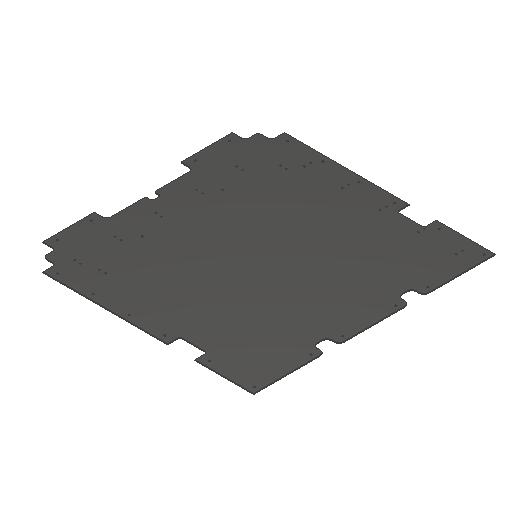
# Autodesk Inventor part: LC_PLEXI_2mm_Side_Wall_Back
Saved by Autodesk Inventor 2026.1 (Build 301233000, 233)
## iProperties
Created: 2016-06-26
Part Number: LC_PLEXI_2mm_Side_Wall_Back
Material: Ogólny
Document SubType Name: Modeling
Designer: Andrzej
Density: 1 g/cm^3
Appearance: Smooth - Black
Mass: 602.344 g
Surface Area: 6069.03 cm^2
Volume: 602.344 cm^3
Author: Andrzej
Autodesk Inventor part; units mm, degrees
ref_plane "YZ Plane" through (0, 0, 0) normal (1, 0, 0) x (0, 1, 0)
ref_plane "XZ Plane" through (0, 0, 0) normal (0, 1, 0) x (-1, 0, 0)
ref_plane "XY Plane" through (0, 0, 0) normal (0, 0, 1) x (1, 0, 0)
sketch "Szkic1" plane through (0, 0, 0) normal (0, 0, 1) x (1, 0, 0)
  line L0 (4.403, -85.7889) -> (549.403, -85.7889)
  line L1 (549.403, -85.7889) -> (549.403, -641.7889)
  line L2 (549.403, -641.7889) -> (4.403, -641.7889)
  line L3 (4.403, -641.7889) -> (4.403, -85.7889)
  line L4 (549.403, -477.9559) -> (521.403, -477.9559)
  line L5 (521.403, -477.9559) -> (521.403, -444.9559)
  line L6 (521.403, -444.9559) -> (549.403, -444.9559)
  line L7 (549.403, -444.9559) -> (549.403, -477.9559)
  line L8 (549.403, -282.6219) -> (521.403, -282.6219)
  line L9 (521.403, -282.6219) -> (521.403, -249.6219)
  line L10 (521.403, -249.6219) -> (549.403, -249.6219)
  line L11 (549.403, -249.6219) -> (549.403, -282.6219)
  line L12 (64.403, -641.7889) -> (64.403, -611.7889)
  line L13 (64.403, -611.7889) -> (34.403, -611.7889)
  line L14 (34.403, -611.7889) -> (34.403, -581.7889)
  line L15 (34.403, -581.7889) -> (4.403, -581.7889)
  line L16 (4.403, -145.7889) -> (34.403, -145.7889)
  line L17 (34.403, -145.7889) -> (34.403, -115.7889)
  line L18 (34.403, -115.7889) -> (64.403, -115.7889)
  line L19 (64.403, -115.7889) -> (64.403, -85.7889)
  line L20 (351.403, -641.7889) -> (414.403, -641.7889)
  line L21 (414.403, -641.7889) -> (414.403, -613.2889)
  line L22 (414.403, -613.2889) -> (351.403, -613.2889)
  line L23 (351.403, -613.2889) -> (351.403, -641.7889)
  line L24 (351.403, -85.7889) -> (414.403, -85.7889)
  line L25 (414.403, -85.7889) -> (414.403, -114.2889)
  line L26 (414.403, -114.2889) -> (351.403, -114.2889)
  line L27 (351.403, -114.2889) -> (351.403, -85.7889)
  line L28 (4.403, -463.7889) -> (32.903, -463.7889)
  line L29 (32.903, -463.7889) -> (32.903, -263.7889)
  line L30 (32.903, -263.7889) -> (4.403, -263.7889)
  line L31 (4.403, -263.7889) -> (4.403, -463.7889)
  line L32 (631.7363, -282.6219) -> (603.7363, -282.6219)
  line L33 (714.0696, -282.6219) -> (686.0696, -282.6219)
  line L34 (32.903, -373.7889) -> (47.903, -373.7889)
  line L35 (47.903, -373.7889) -> (47.903, -353.7889)
  line L36 (47.903, -353.7889) -> (32.903, -353.7889)
  point P0 (0, 0)
  point P1 (331.403, -628.2889)
  point P2 (84.403, -628.2889)
  point P3 (84.403, -99.2889)
  point P4 (331.403, -99.2889)
  point P5 (537.903, -628.2889)
  point P6 (434.403, -628.2889)
  point P7 (537.903, -497.9559)
  point P8 (537.903, -424.9559)
  point P9 (537.903, -302.6219)
  point P10 (537.903, -229.6219)
  point P11 (537.903, -99.2889)
  point P12 (434.403, -99.2889)
  point P13 (17.903, -561.7889)
  point P14 (17.903, -483.7889)
  point P15 (17.903, -243.7889)
  point P16 (17.903, -165.7889)
  point P17 (166.7363, -628.2889)
  point P18 (249.0696, -628.2889)
  point P19 (166.7363, -99.2889)
  point P20 (249.0696, -99.2889)
  point P21 (107.903, -456.4556)
  point P22 (107.903, -271.1223)
  dimension "d0" = 545
  dimension "d1" = 556
  dimension "d4" = 28
  dimension "d5" = 33
  dimension "d6" = 28
  dimension "d7" = 33
  dimension "d8" = 163.833
  dimension "d9" = 163.833
  dimension "d13" = 30
  dimension "d14" = 30
  dimension "d15" = 30
  dimension "d16" = 30
  dimension "d17" = 30
  dimension "d18" = 30
  dimension "d19" = 30
  dimension "d20" = 30
  dimension "d22" = 63
  dimension "d23" = 28.5
  dimension "d24" = 63
  dimension "d25" = 28.5
  dimension "d26" = 347
  dimension "d27" = 347
  dimension "d29" = 28.5
  dimension "d30" = 200
  dimension "d31" = 178
  dimension "d33" = 20
  dimension "d34" = 13.5
  dimension "d35" = 13.5
  dimension "d36" = 13.5
  dimension "d37" = 13.5
  dimension "d38" = 11.5
  dimension "d39" = 11.5
  dimension "d40" = 11.5
  dimension "d41" = 11.5
  dimension "d42" = 11.5
  dimension "d43" = 11.5
  dimension "d44" = 13.5
  dimension "d45" = 13.5
  dimension "d46" = 13.5
  dimension "d47" = 13.5
  dimension "d48" = 13.5
  dimension "d49" = 13.5
  dimension "d50" = 13.5
  dimension "d51" = 13.5
  dimension "d52" = 20
  dimension "d53" = 20
  dimension "d54" = 20
  dimension "d55" = 20
  dimension "d56" = 20
  dimension "d57" = 20
  dimension "d58" = 20
  dimension "d59" = 20
  dimension "d60" = 20
  dimension "d61" = 20
  dimension "d62" = 20
  dimension "d63" = 20
  dimension "d64" = 20
  dimension "d65" = 247
  dimension "d68" = 82.3333
  dimension "d75" = 82.3333
  dimension "d87" = 103.5
  dimension "d88" = 103.5
  dimension "d89" = 185.3333
  dimension "d90" = 185.3333
  constraints: 74 end point, 14 perpendicular, 12 parallel, 11 point on line, 10 horizontal, 1 vertical, 10 other
  measures "d0" distance of L1.end L2.end
  measures "d1" distance of L0.end L1.end
  measures "d4" distance of L5.end L6.end
  measures "d5" distance of L4.end L5.end
  measures "d6" distance of L9.end L10.end
  measures "d7" distance of L8.end L9.end
  measures "d8" distance between parallel lines of L2 L4
  measures "d9" distance between parallel lines of L0 L10
  measures "d13" distance of L12.start L12.end
  measures "d14" distance of L12.end L13.end
  measures "d15" distance of L13.end L14.end
  measures "d16" distance of L14.end L15.end
  measures "d17" distance of L16.start L16.end
  measures "d18" distance of L16.end L17.end
  measures "d19" distance of L17.end L18.end
  measures "d20" distance of L18.end L19.end
  measures "d22" distance between parallel lines of L21 L23
  measures "d23" distance between parallel lines of L20 L22
  measures "d24" distance of L25.end L26.end
  measures "d25" distance of L24.end L25.end
  measures "d26" distance between parallel lines of L3 L23
  measures "d27" distance between parallel lines of L3 L27
  measures "d29" distance of L30.end L29.end
  measures "d30" distance of L29.end L28.end
  measures "d31" distance between parallel lines of L2 L28
  measures "d33" distance from line of L12 point (84.403, -628.289)
  measures "d34" distance from line of L2 point (84.403, -628.289)
  measures "d35" distance from line of L2 point (331.403, -628.289)
  measures "d36" distance from line of L2 point (434.403, -628.289)
  measures "d37" distance from line of L2 point (537.903, -628.289)
  measures "d38" distance from line of L1 point (537.903, -628.289)
  measures "d39" distance from line of L1 point (537.903, -497.956)
  measures "d40" distance from line of L1 point (537.903, -424.956)
  measures "d41" distance from line of L1 point (537.903, -302.622)
  measures "d42" distance from line of L1 point (537.903, -229.622)
  measures "d43" distance from line of L1 point (537.903, -99.289)
  measures "d44" distance from line of L0 point (537.903, -99.289)
  measures "d45" distance from line of L0 point (434.403, -99.289)
  measures "d46" distance from line of L0 point (331.403, -99.289)
  measures "d47" distance from line of L0 point (84.403, -99.289)
  measures "d48" distance from line of L3 point (17.903, -165.789)
  measures "d49" distance from line of L3 point (17.903, -243.789)
  measures "d50" distance from line of L3 point (17.903, -483.789)
  measures "d51" distance from line of L3 point (17.903, -561.789)
  measures "d52" distance from line of L28 point (17.903, -483.789)
  measures "d53" distance from line of L15 point (17.903, -561.789)
  measures "d54" distance from line of L30 point (17.903, -243.789)
  measures "d55" distance from line of L16 point (17.903, -165.789)
  measures "d56" distance from line of L19 point (84.403, -99.289)
  measures "d57" distance from line of L27 point (331.403, -99.289)
  measures "d58" distance from line of L25 point (434.403, -99.289)
  measures "d59" distance from line of L10 point (537.903, -229.622)
  measures "d60" distance from line of L8 point (537.903, -302.622)
  measures "d61" distance from line of L6 point (537.903, -424.956)
  measures "d62" distance from line of L4 point (537.903, -497.956)
  measures "d63" distance from line of L21 point (434.403, -628.289)
  measures "d64" distance from line of L23 point (331.403, -628.289)
  measures "d65" distance of point (331.403, -628.289) point (84.403, -628.289)
  measures "d68" distance of L8.start L32.start
  measures "d75" distance of point (84.403, -99.289) point (166.736, -99.289)
  measures "d87" distance from line of point (107.903, -456.456) L3
  measures "d88" distance from line of L3 point (107.903, -271.122)
  measures "d89" distance from line of L2 point (107.903, -456.456)
  measures "d90" distance from line of L0 point (107.903, -271.122)
extrude "Wyciągnięcie proste1" add sketch "Szkic1" along normal blind 2
extrude "Wyciągnięcie proste2" cut sketch "Szkic1" along normal blind 2 contours L0 L19 L18 L17 L16 L3 | L0 L25 L26 L27 | L30 L29 L28 L3 | L15 L14 L13 L12 L2 L3 | L36 L35 L34 L29 | L1 L8 L9 L10 | L1 L4 L5 L6 | L23 L22 L21 L2
fillet "Zaokrąglenie1" radius 10 8 edges at (549.403, -477.9559, 1) (521.403, -477.9559, 1) (521.403, -444.9559, 1) (549.403, -444.9559, 1) (549.403, -282.6219, 1) (521.403, -282.6219, 1) (521.403, -249.6219, 1) (549.403, -249.6219, 1)
fillet "Zaokrąglenie2" radius 8 6 edges at (34.403, -581.7889, 1) (34.403, -611.7889, 1) (64.403, -611.7889, 1) (34.403, -145.7889, 1) (34.403, -115.7889, 1) (64.403, -115.7889, 1)
fillet "Zaokrąglenie3" radius 5 4 edges at (351.403, -613.2889, 1) (414.403, -613.2889, 1) (351.403, -114.2889, 1) (414.403, -114.2889, 1)
fillet "Zaokrąglenie4" radius 10 2 edges at (32.903, -463.7889, 1) (32.903, -263.7889, 1)
hole "Otwór1" at (331.403, -628.2889, 0) at (84.403, -628.2889, 0) at (84.403, -99.2889, 0) at (331.403, -99.2889, 0) at (537.903, -628.2889, 0) at (434.403, -628.2889, 0) at (537.903, -497.9559, 0) at (537.903, -424.9559, 0) at (537.903, -302.6219, 0) at (537.903, -229.6219, 0) at (537.903, -99.2889, 0) at (434.403, -99.2889, 0) at (17.903, -561.7889, 0) at (17.903, -483.7889, 0) at (17.903, -243.7889, 0) at (17.903, -165.7889, 0) at (166.7363, -628.2889, 0) at (249.0696, -628.2889, 0) at (166.7363, -99.2889, 0) at (249.0696, -99.2889, 0) at (107.903, -456.4556, 0) at (107.903, -271.1223, 0) direction (0, 0, 1) diameter 4 end through all
fillet "Zaokrąglenie5" radius 4 4 edges at (32.903, -373.7889, 1) (47.903, -373.7889, 1) (47.903, -353.7889, 1) (32.903, -353.7889, 1)
sketch "Szkic2" plane through (0, 0, 0) normal (0, 0, -1) x (-1, 0, 0)
  circle A0 centre (-107.903, -456.4556) radius 2 projected
  circle A1 centre (-166.7363, -99.2889) radius 2 projected
  circle A2 centre (-166.7363, -628.2889) radius 2 projected
  circle A3 centre (-17.903, -243.7889) radius 2 projected
  circle A4 centre (-17.903, -561.7889) radius 2 projected
  circle A5 centre (-537.903, -99.2889) radius 2 projected
  circle A6 centre (-537.903, -302.6219) radius 2 projected
  circle A7 centre (-537.903, -497.9559) radius 2 projected
  circle A8 centre (-537.903, -628.2889) radius 2 projected
  circle A9 centre (-84.403, -99.2889) radius 2 projected
  circle A10 centre (-331.403, -628.2889) radius 2 projected
  circle A11 centre (-84.403, -628.2889) radius 2 projected
  circle A12 centre (-331.403, -99.2889) radius 2 projected
  circle A13 centre (-434.403, -628.2889) radius 2 projected
  circle A14 centre (-537.903, -424.9559) radius 2 projected
  circle A15 centre (-537.903, -229.6219) radius 2 projected
  circle A16 centre (-434.403, -99.2889) radius 2 projected
  circle A17 centre (-17.903, -483.7889) radius 2 projected
  circle A18 centre (-17.903, -165.7889) radius 2 projected
  circle A19 centre (-249.0696, -628.2889) radius 2 projected
  circle A20 centre (-249.0696, -99.2889) radius 2 projected
  circle A21 centre (-107.903, -271.1223) radius 2 projected
  arc A22 (-36.903, -353.7889) -> (-32.903, -349.7889) centre (-36.903, -349.7889) ccw projected
  line L0 (-32.903, -349.7889) -> (-32.903, -273.7889) projected
  arc A23 (-22.903, -263.7889) -> (-32.903, -273.7889) centre (-22.903, -273.7889) ccw projected
  line L1 (-22.903, -263.7889) -> (-4.403, -263.7889) projected
  line L2 (-4.403, -263.7889) -> (-4.403, -145.7889) projected
  line L3 (-4.403, -145.7889) -> (-26.403, -145.7889) projected
  arc A24 (-34.403, -137.7889) -> (-26.403, -145.7889) centre (-26.403, -137.7889) ccw projected
  line L4 (-34.403, -137.7889) -> (-34.403, -123.7889) projected
  arc A25 (-34.403, -123.7889) -> (-42.403, -115.7889) centre (-42.403, -123.7889) ccw projected
  line L5 (-42.403, -115.7889) -> (-56.403, -115.7889) projected
  arc A26 (-64.403, -107.7889) -> (-56.403, -115.7889) centre (-56.403, -107.7889) ccw projected
  line L6 (-64.403, -107.7889) -> (-64.403, -85.7889) projected
  line L7 (-64.403, -85.7889) -> (-351.403, -85.7889) projected
  line L8 (-351.403, -85.7889) -> (-351.403, -109.2889) projected
  arc A27 (-356.403, -114.2889) -> (-351.403, -109.2889) centre (-356.403, -109.2889) ccw projected
  line L9 (-356.403, -114.2889) -> (-409.403, -114.2889) projected
  arc A28 (-414.403, -109.2889) -> (-409.403, -114.2889) centre (-409.403, -109.2889) ccw projected
  line L10 (-414.403, -109.2889) -> (-414.403, -85.7889) projected
  line L11 (-414.403, -85.7889) -> (-549.403, -85.7889) projected
  line L12 (-549.403, -85.7889) -> (-549.403, -239.6219) projected
  arc A29 (-549.403, -239.6219) -> (-539.403, -249.6219) centre (-539.403, -239.6219) ccw projected
  line L13 (-539.403, -249.6219) -> (-531.403, -249.6219) projected
  arc A30 (-521.403, -259.6219) -> (-531.403, -249.6219) centre (-531.403, -259.6219) ccw projected
  line L14 (-521.403, -259.6219) -> (-521.403, -272.6219) projected
  arc A31 (-531.403, -282.6219) -> (-521.403, -272.6219) centre (-531.403, -272.6219) ccw projected
  line L15 (-531.403, -282.6219) -> (-539.403, -282.6219) projected
  arc A32 (-539.403, -282.6219) -> (-549.403, -292.6219) centre (-539.403, -292.6219) ccw projected
  line L16 (-549.403, -292.6219) -> (-549.403, -434.9559) projected
  arc A33 (-549.403, -434.9559) -> (-539.403, -444.9559) centre (-539.403, -434.9559) ccw projected
  line L17 (-539.403, -444.9559) -> (-531.403, -444.9559) projected
  arc A34 (-521.403, -454.9559) -> (-531.403, -444.9559) centre (-531.403, -454.9559) ccw projected
  line L18 (-521.403, -454.9559) -> (-521.403, -467.9559) projected
  arc A35 (-531.403, -477.9559) -> (-521.403, -467.9559) centre (-531.403, -467.9559) ccw projected
  line L19 (-531.403, -477.9559) -> (-539.403, -477.9559) projected
  arc A36 (-539.403, -477.9559) -> (-549.403, -487.9559) centre (-539.403, -487.9559) ccw projected
  line L20 (-549.403, -487.9559) -> (-549.403, -641.7889) projected
  line L21 (-549.403, -641.7889) -> (-414.403, -641.7889) projected
  line L22 (-414.403, -641.7889) -> (-414.403, -618.2889) projected
  arc A37 (-409.403, -613.2889) -> (-414.403, -618.2889) centre (-409.403, -618.2889) ccw projected
  line L23 (-409.403, -613.2889) -> (-356.403, -613.2889) projected
  arc A38 (-351.403, -618.2889) -> (-356.403, -613.2889) centre (-356.403, -618.2889) ccw projected
  line L24 (-351.403, -618.2889) -> (-351.403, -641.7889) projected
  line L25 (-351.403, -641.7889) -> (-64.403, -641.7889) projected
  line L26 (-64.403, -641.7889) -> (-64.403, -619.7889) projected
  arc A39 (-56.403, -611.7889) -> (-64.403, -619.7889) centre (-56.403, -619.7889) ccw projected
  line L27 (-56.403, -611.7889) -> (-42.403, -611.7889) projected
  arc A40 (-42.403, -611.7889) -> (-34.403, -603.7889) centre (-42.403, -603.7889) ccw projected
  line L28 (-34.403, -603.7889) -> (-34.403, -589.7889) projected
  arc A41 (-26.403, -581.7889) -> (-34.403, -589.7889) centre (-26.403, -589.7889) ccw projected
  line L29 (-26.403, -581.7889) -> (-4.403, -581.7889) projected
  line L30 (-4.403, -581.7889) -> (-4.403, -463.7889) projected
  line L31 (-4.403, -463.7889) -> (-22.903, -463.7889) projected
  arc A42 (-32.903, -453.7889) -> (-22.903, -463.7889) centre (-22.903, -453.7889) ccw projected
  line L32 (-32.903, -453.7889) -> (-32.903, -377.7889) projected
  arc A43 (-32.903, -377.7889) -> (-36.903, -373.7889) centre (-36.903, -377.7889) ccw projected
  line L33 (-36.903, -373.7889) -> (-43.903, -373.7889) projected
  arc A44 (-47.903, -369.7889) -> (-43.903, -373.7889) centre (-43.903, -369.7889) ccw projected
  line L34 (-47.903, -369.7889) -> (-47.903, -357.7889) projected
  arc A45 (-43.903, -353.7889) -> (-47.903, -357.7889) centre (-43.903, -357.7889) ccw projected
  line L35 (-43.903, -353.7889) -> (-36.903, -353.7889) projected
  line L36 (-615.8075, -114.2889) -> (87.7872, -114.2889)
  line L37 (87.7872, -613.2889) -> (-656.0971, -613.2889)
  line L38 (-32.903, -1298.7414) -> (-32.903, 136.0464)
  line L39 (-92.903, 107.9926) -> (-92.903, -1119.5481)
  line L40 (-122.903, 112.1333) -> (-122.903, -1130.021)
  line L41 (-75.903, -580.2889) -> (-77.903, -580.2889)
  line L42 (-77.903, -580.2889) -> (-77.903, -583.2889)
  line L43 (-77.903, -583.2889) -> (-75.903, -583.2889)
  line L44 (-75.903, -583.2889) -> (-75.903, -580.2889)
  line L45 (-89.903, -580.2889) -> (-91.903, -580.2889)
  line L46 (-91.903, -580.2889) -> (-91.903, -583.2889)
  line L47 (-91.903, -583.2889) -> (-89.903, -583.2889)
  line L48 (-89.903, -583.2889) -> (-89.903, -580.2889)
  line L49 (-77.903, -489.7889) -> (-75.903, -489.7889)
  line L50 (-89.903, -489.7889) -> (-89.903, -486.7889)
  line L51 (-75.903, -486.7889) -> (-77.903, -486.7889)
  line L52 (-75.903, -489.7889) -> (-75.903, -486.7889)
  line L53 (-77.903, -486.7889) -> (-77.903, -489.7889)
  line L54 (-91.903, -489.7889) -> (-89.903, -489.7889)
  line L55 (-89.903, -486.7889) -> (-91.903, -486.7889)
  line L56 (-91.903, -486.7889) -> (-91.903, -489.7889)
  line L57 (-77.903, -396.2889) -> (-75.903, -396.2889)
  line L58 (-89.903, -396.2889) -> (-89.903, -393.2889)
  line L59 (-75.903, -393.2889) -> (-77.903, -393.2889)
  line L60 (-75.903, -396.2889) -> (-75.903, -393.2889)
  line L61 (-77.903, -393.2889) -> (-77.903, -396.2889)
  line L62 (-91.903, -396.2889) -> (-89.903, -396.2889)
  line L63 (-89.903, -393.2889) -> (-91.903, -393.2889)
  line L64 (-91.903, -393.2889) -> (-91.903, -396.2889)
  line L65 (-77.903, -302.7889) -> (-75.903, -302.7889)
  line L66 (-89.903, -302.7889) -> (-89.903, -299.7889)
  line L67 (-75.903, -299.7889) -> (-77.903, -299.7889)
  line L68 (-75.903, -302.7889) -> (-75.903, -299.7889)
  line L69 (-77.903, -299.7889) -> (-77.903, -302.7889)
  line L70 (-91.903, -302.7889) -> (-89.903, -302.7889)
  line L71 (-89.903, -299.7889) -> (-91.903, -299.7889)
  line L72 (-91.903, -299.7889) -> (-91.903, -302.7889)
  line L73 (-77.903, -209.2889) -> (-75.903, -209.2889)
  line L74 (-89.903, -209.2889) -> (-89.903, -206.2889)
  line L75 (-75.903, -206.2889) -> (-77.903, -206.2889)
  line L76 (-75.903, -209.2889) -> (-75.903, -206.2889)
  line L77 (-77.903, -206.2889) -> (-77.903, -209.2889)
  line L78 (-91.903, -209.2889) -> (-89.903, -209.2889)
  line L79 (-89.903, -206.2889) -> (-91.903, -206.2889)
  line L80 (-91.903, -206.2889) -> (-91.903, -209.2889)
  line L81 (-123.903, -154.2889) -> (-125.903, -154.2889)
  line L82 (-125.903, -154.2889) -> (-125.903, -157.2889)
  line L83 (-125.903, -157.2889) -> (-123.903, -157.2889)
  line L84 (-123.903, -157.2889) -> (-123.903, -154.2889)
  line L85 (-137.903, -157.2889) -> (-137.903, -154.2889)
  line L86 (-139.903, -154.2889) -> (-139.903, -157.2889)
  line L87 (-137.903, -154.2889) -> (-139.903, -154.2889)
  line L88 (-139.903, -157.2889) -> (-137.903, -157.2889)
  line L89 (-152.903, -131.2889) -> (-152.903, -129.2889)
  line L90 (-152.903, -129.2889) -> (-155.903, -129.2889)
  line L91 (-155.903, -129.2889) -> (-155.903, -131.2889)
  line L92 (-155.903, -131.2889) -> (-152.903, -131.2889)
  line L93 (-155.903, -117.2889) -> (-152.903, -117.2889)
  line L94 (-152.903, -115.2889) -> (-155.903, -115.2889)
  line L95 (-152.903, -117.2889) -> (-152.903, -115.2889)
  line L96 (-155.903, -115.2889) -> (-155.903, -117.2889)
  line L97 (-522.903, -793.5425) -> (-522.903, 26.7944)
  line L98 (-240.403, -131.2889) -> (-240.403, -129.2889)
  line L99 (-243.403, -129.2889) -> (-243.403, -131.2889)
  line L100 (-240.403, -117.2889) -> (-240.403, -115.2889)
  line L101 (-240.403, -115.2889) -> (-243.403, -115.2889)
  line L102 (-243.403, -131.2889) -> (-240.403, -131.2889)
  line L103 (-240.403, -129.2889) -> (-243.403, -129.2889)
  line L104 (-243.403, -115.2889) -> (-243.403, -117.2889)
  line L105 (-243.403, -117.2889) -> (-240.403, -117.2889)
  line L106 (-327.903, -131.2889) -> (-327.903, -129.2889)
  line L107 (-330.903, -129.2889) -> (-330.903, -131.2889)
  line L108 (-327.903, -117.2889) -> (-327.903, -115.2889)
  line L109 (-327.903, -115.2889) -> (-330.903, -115.2889)
  line L110 (-330.903, -131.2889) -> (-327.903, -131.2889)
  line L111 (-327.903, -129.2889) -> (-330.903, -129.2889)
  line L112 (-330.903, -115.2889) -> (-330.903, -117.2889)
  line L113 (-330.903, -117.2889) -> (-327.903, -117.2889)
  line L114 (-415.403, -131.2889) -> (-415.403, -129.2889)
  line L115 (-418.403, -129.2889) -> (-418.403, -131.2889)
  line L116 (-415.403, -117.2889) -> (-415.403, -115.2889)
  line L117 (-415.403, -115.2889) -> (-418.403, -115.2889)
  line L118 (-418.403, -131.2889) -> (-415.403, -131.2889)
  line L119 (-415.403, -129.2889) -> (-418.403, -129.2889)
  line L120 (-418.403, -115.2889) -> (-418.403, -117.2889)
  line L121 (-418.403, -117.2889) -> (-415.403, -117.2889)
  line L122 (-502.903, -131.2889) -> (-502.903, -129.2889)
  line L123 (-505.903, -129.2889) -> (-505.903, -131.2889)
  line L124 (-502.903, -117.2889) -> (-502.903, -115.2889)
  line L125 (-502.903, -115.2889) -> (-505.903, -115.2889)
  line L126 (-505.903, -131.2889) -> (-502.903, -131.2889)
  line L127 (-502.903, -129.2889) -> (-505.903, -129.2889)
  line L128 (-505.903, -115.2889) -> (-505.903, -117.2889)
  line L129 (-505.903, -117.2889) -> (-502.903, -117.2889)
  line L130 (-123.903, -570.2889) -> (-125.903, -570.2889)
  line L131 (-125.903, -570.2889) -> (-125.903, -573.2889)
  line L132 (-125.903, -573.2889) -> (-123.903, -573.2889)
  line L133 (-123.903, -573.2889) -> (-123.903, -570.2889)
  line L134 (-137.903, -573.2889) -> (-137.903, -570.2889)
  line L135 (-139.903, -570.2889) -> (-139.903, -573.2889)
  line L136 (-137.903, -570.2889) -> (-139.903, -570.2889)
  line L137 (-139.903, -573.2889) -> (-137.903, -573.2889)
  point P0 (0, 0)
  point P1 (-81.6253, -209.2889)
  point P2 (-502.903, -149.0443)
  dimension "d95" = 28.5
  dimension "d96" = 28.5
  dimension "d97" = 28.5
  dimension "d98" = 30
  dimension "d99" = 15
  dimension "d100" = 2
  dimension "d101" = 3
  dimension "d102" = 2
  dimension "d103" = 3
  dimension "d104" = 12
  dimension "d105" = 1
  dimension "d106" = 30
  dimension "d107" = 95
  dimension "d108" = 374
  dimension "d111" = 93.5
  dimension "d120" = 2
  dimension "d121" = 3
  dimension "d122" = 2
  dimension "d123" = 3
  dimension "d124" = 12
  dimension "d125" = 1
  dimension "d126" = 40
  dimension "d133" = 2
  dimension "d134" = 3
  dimension "d135" = 2
  dimension "d136" = 3
  dimension "d137" = 12
  dimension "d140" = 30
  dimension "d141" = 1
  dimension "d142" = 26.5
  dimension "d143" = 20
  dimension "d144" = 350
  dimension "d147" = 87.5
  dimension "d160" = 2
  dimension "d161" = 3
  dimension "d162" = 2
  dimension "d163" = 3
  dimension "d164" = 12
  dimension "d166" = 40
  dimension "d167" = 1
  constraints: 204 end point, 17 parallel, 9 horizontal, 8 perpendicular, 5 vertical, 4 collinear, 128 other
  measures "d95" distance between parallel lines of L7 L36
  measures "d96" distance between parallel lines of L25 L37
  measures "d97" distance between parallel lines of L2 L38
  measures "d98" distance between parallel lines of L40 L39
  measures "d99" distance from line of L39 A21.centre
  measures "d100" distance of L43.end L42.end
  measures "d101" distance of L42.end L41.end
  measures "d102" distance of L48.start L46.end
  measures "d103" distance of L46.end L46.start
  measures "d104" distance between parallel lines of L48 L42
  measures "d105" distance between parallel lines of L39 L46
  measures "d106" distance between parallel lines of L37 L47
  measures "d107" distance from line of L36 point (-81.625, -209.289)
  measures "d108" distance from line of L43 point (-81.625, -209.289)
  measures "d111" distance of L42.end L49.start
  measures "d120" distance of L83.end L82.end
  measures "d121" distance of L82.end L81.end
  measures "d122" distance of L85.start L86.end
  measures "d123" distance of L86.end L86.start
  measures "d124" distance between parallel lines of L85 L82
  measures "d125" distance from line of L40 L83.end
  measures "d126" distance between parallel lines of L36 L81
  measures "d133" distance of L91.end L91.start
  measures "d134" distance of L91.start L89.end
  measures "d135" distance of L96.end L96.start
  measures "d136" distance of L96.start L94.start
  measures "d137" distance between parallel lines of L93 L90
  measures "d140" distance between parallel lines of L40 L95
  measures "d141" distance between parallel lines of L36 L94
  measures "d142" distance between parallel lines of L12 L97
  measures "d143" distance from line of L97 point (-502.903, -149.044)
  measures "d144" distance from line of point (-502.903, -149.044) L89
  measures "d147" distance of L92.end L98.start
  measures "d160" distance of L133.start L131.end
  measures "d161" distance of L131.end L130.end
  measures "d162" distance of L137.end L137.start
  measures "d163" distance of L137.start L135.start
  measures "d164" distance between parallel lines of L134 L131
  measures "d166" distance between parallel lines of L37 L132
  measures "d167" distance between parallel lines of L40 L133
extrude "Wyciągnięcie proste3" cut sketch "Szkic2" against normal through all contours L44 L43 L42 L41 | L48 L47 L46 L45 | L53 L51 L52 L49 | L54 L56 L55 L50 | L61 L59 L60 L57 | L62 L64 L63 L58 | L69 L67 L68 L65 | L70 L72 L71 L66 | L77 L75 L76 L73 | L78 L80 L79 L74 | L84 L83 L82 L81 | L88 L86 L87 L85 | L92 L91 L90 L89 | L96 L94 L95 L93 | L102 L99 L103 L98 | L105 L104 L101 L100 | L110 L107 L111 L106 | L113 L112 L109 L108 | L118 L115 L119 L114 | L121 L120 L117 L116 | L126 L123 L127 L122 | L129 L128 L125 L124 | L133 L132 L131 L130 | L137 L135 L136 L134
equation "\"d4\" = d6"
equation "\"d9\" = d8"
equation "\"d24\" = d22"
equation "\"d25\" = d23"
equation "\"d27\" = d26"
equation "\"d31\" = -0.5 * d30 + 0.5 * d1"
equation "\"d39\" = d38"
equation "\"d40\" = d38"
equation "\"d41\" = d38"
equation "\"d42\" = d38"
equation "\"d43\" = d38"
equation "\"d88\" = d87"
equation "\"d124\" = d104"
